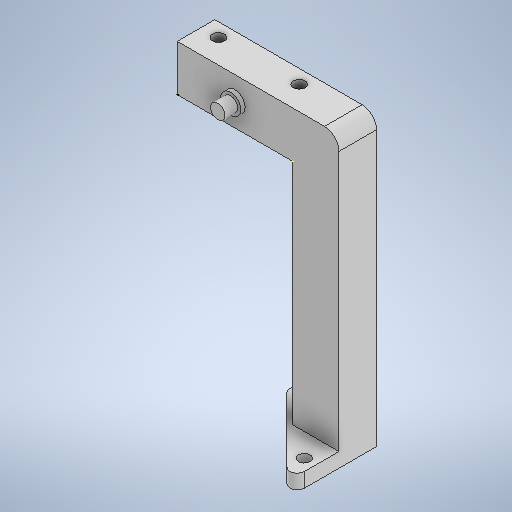
# Autodesk Inventor part: 13042026-06
Saved by Autodesk Inventor 2025.2 (Build 292293000, 293)
## iProperties
Created: 2026-05-05
Part Number: 13042026-06
Material: Generic
Document SubType Name: Modeling
Designer: Oski
Density: 1 g/cm^3
Appearance: Default
Author: Oski
Autodesk Inventor part; units mm, degrees
ref_plane "YZ Plane" through (0, 0, 0) normal (1, 0, 0) x (0, 1, 0)
ref_plane "XZ Plane" through (0, 0, 0) normal (0, 1, 0) x (-1, 0, 0)
ref_plane "XY Plane" through (0, 0, 0) normal (0, 0, 1) x (1, 0, 0)
sketch "Sketch2" plane through (0, 0, 0) normal (0, 0, 1) x (1, 0, 0)
  line L0 (-40, 16) -> (40, 16)
  line L1 (40, 16) -> (40, -16)
  line L2 (40, -16) -> (-40, -16)
  line L3 (-40, -16) -> (-40, 16)
  line L4 (-40, 16) -> (40, -16) construction
  line L5 (40, 16) -> (-40, -16) construction
  point P0 (0, 0)
  dimension "d4" = 32
  dimension "d5" = 80
  constraints: 12 end point, 2 midpoint, 2 parallel, 1 horizontal, 1 perpendicular
  measures "d4" distance of L0.end L1.end
  measures "d5" distance of L1.end L2.end
extrude "Extrusion1" add sketch "Sketch2" along normal blind 26
sketch "Sketch3" plane through (0, 0, 26) normal (0, 0, 1) x (1, 0, 0)
  circle A0 centre (0, 0) radius 7
  dimension "d8" = 14
  constraints: 1 centre point, 1 coincident
  measures "d8" diameter of A0
extrude "Extrusion2" add sketch "Sketch3" along normal blind 3
sketch "Sketch4" plane through (0, 0, 29) normal (0, 0, 1) x (1, 0, 0)
  circle A0 centre (0, 0) radius 4.95
  dimension "d11" = 9.9
  constraints: 1 centre point, 1 coincident
  measures "d11" diameter of A0
extrude "Extrusion3" add sketch "Sketch4" along normal blind 9
sketch "Sketch6" plane through (-40, 16, 0) normal (0, 1, 0) x (1, 0, 0)
  line L0 (12, -9.5) -> (0, -9.5) construction
  line L1 (0, 0) -> (0, -26) projected
  line L2 (68, -9.5) -> (80, -9.5) construction
  line L3 (80, 0) -> (80, -26) projected
  line L4 (80, 0) -> (0, 0) projected
  point P0 (40, 0)
  point P1 (74, -9.5)
  dimension "d29" = 56
  dimension "d30" = 9.5
  constraints: 4 end point, 3 point on line, 2 horizontal, 1 collinear, 1 midpoint
  measures "d29" distance of L2.start L0.start
  measures "d30" distance from line of L4 point (74, -9.5)
hole "Hole3" at (-28, 16, 9.5) at (28, 16, 9.5) direction (0, -1, 0) diameter 8.3 end through all
sketch "Sketch7" plane through (-40, -16, 0) normal (0, -1, 0) x (1, 0, 0)
  line L0 (80, 0) -> (80, 26) projected
  line L1 (0, 0) -> (0, 26) projected
  line L2 (80, 0) -> (0, 26)
  point P0 (40, 0)
  constraints: 2 end point
sketch "Sketch9" plane through (40, -16, 0) normal (1, 0, 0) x (0, 0, -1)
  line L0 (0, 0) -> (0, 32) projected
  line L1 (0, 32) -> (-26, 32)
  line L2 (-26, 32) -> (-26, -168)
  line L3 (-26, -168) -> (0, -168)
  line L4 (0, -168) -> (0, 32)
  line L5 (-26, 0) -> (-26, 32) projected
  point P0 (0, 16)
  dimension "d38" = 200
  constraints: 8 end point, 2 parallel, 1 horizontal, 1 perpendicular, 1 point on line
  measures "d38" distance of L3.end L0.end
extrude "Extrusion4" add sketch "Sketch9" along normal blind 32
sketch "Sketch11" plane through (40, -184, 0) normal (0, -1, 0) x (1, 0, 0)
  line L0 (32, 0) -> (-30, 0)
  line L1 (32, 62) -> (-30, 0)
  line L2 (32, 0) -> (32, 62)
  point P0 (-40, 0)
  point P1 (0, 0)
  dimension "d43" = 62
  dimension "d44" = 62
  constraints: 7 end point, 1 perpendicular, 1 point on line
  measures "d43" distance of L0.start L1.start
  measures "d44" distance of L0.start L0.end
extrude "Extrusion5" add sketch "Sketch11" against normal blind 10
fillet "Fillet1" radius 5 2 edges at (10, -179, 0) (72, -179, 62)
sketch "Sketch12" plane through (72, -184, 0) normal (0, -1, 0) x (1, 0, 0)
  line L0 (0, 0) -> (-32, 0)
  line L1 (-32, 0) -> (-32, 32)
  line L2 (-32, 32) -> (0, 32)
  line L3 (0, 32) -> (0, 0)
  circle A0 centre (-44, 9.5) radius 4.15 projected
  line L4 (-49.9289, 0) -> (0, 0) projected
  line L5 (0, 0) -> (0, 49.9289) projected
  point P0 (-72, 0)
  point P1 (-8, 42)
  point P2 (-42, 8)
  dimension "d48" = 32
  dimension "d49" = 32
  dimension "d50" = 8
  dimension "d51" = 10
  dimension "d52" = 10
  dimension "d53" = 8
  constraints: 8 end point, 2 parallel, 1 coincident, 1 horizontal, 1 perpendicular
  measures "d48" distance of L1.end L2.end
  measures "d49" distance of L0.end L1.end
  measures "d50" distance from line of L4 point (-42, 8)
  measures "d51" distance from line of L1 point (-42, 8)
  measures "d52" distance from line of L2 point (-8, 42)
  measures "d53" distance from line of L5 point (-8, 42)
hole "Hole4" at (64, -184, 42) at (30, -184, 8) direction (0, 1, 0) diameter 8.2 depth 20
fillet "Fillet2" radius 10 1 edges at (72, 16, 13)
body "Solid1"
